Autodesk Inventor part; units mm, degrees
(part 2 of 3)
  line L954 (15.7927, 2.8054) -> (15.8047, 2.9296)
  line L955 (15.8047, 2.9296) -> (15.8214, 3.0524)
  line L956 (15.8214, 3.0524) -> (15.8318, 3.1132)
  line L957 (15.8318, 3.1132) -> (15.8442, 3.1734)
  line L958 (15.8442, 3.1734) -> (15.5913, 3.315)
  line L959 (15.5913, 3.315) -> (15.2554, 3.4241)
  line L960 (15.2554, 3.4241) -> (14.9676, 3.4583)
  line L961 (14.9676, 3.4583) -> (14.9422, 3.4023)
  line L962 (14.9422, 3.4023) -> (14.915, 3.3469)
  line L963 (14.915, 3.3469) -> (14.8562, 3.2378)
  line L964 (14.8562, 3.2378) -> (14.7929, 3.1303)
  line L965 (14.7929, 3.1303) -> (14.7259, 3.0241)
  line L966 (14.7259, 3.0241) -> (14.5818, 2.8156)
  line L967 (14.5818, 2.8156) -> (14.4261, 2.6115)
  line L968 (14.4261, 2.6115) -> (14.2601, 2.4115)
  line L969 (14.2601, 2.4115) -> (14.0847, 2.2154)
  line L970 (14.0847, 2.2154) -> (13.9004, 2.0233)
  line L971 (13.9004, 2.0233) -> (13.7077, 1.8349)
  line L972 (13.7077, 1.8349) -> (13.507, 1.6503)
  line L973 (13.507, 1.6503) -> (13.3514, 1.5144)
  line L974 (13.3514, 1.5144) -> (12.8549, 1.72)
  line L975 (12.8549, 1.72) -> (12.841, 1.9262)
  line L976 (12.841, 1.9262) -> (12.8296, 2.1986)
  line L977 (12.8296, 2.1986) -> (12.8265, 2.4681)
  line L978 (12.8265, 2.4681) -> (12.8321, 2.7343)
  line L979 (12.8321, 2.7343) -> (12.8466, 2.997)
  line L980 (12.8466, 2.997) -> (12.8707, 3.2557)
  line L981 (12.8707, 3.2557) -> (12.9049, 3.5101)
  line L982 (12.9049, 3.5101) -> (12.9505, 3.7595)
  line L983 (12.9505, 3.7595) -> (12.9781, 3.882)
  line L984 (12.9781, 3.882) -> (13.0095, 4.0027)
  line L985 (13.0095, 4.0027) -> (13.0451, 4.1215)
  line L986 (13.0451, 4.1215) -> (13.0649, 4.1799)
  line L987 (13.0649, 4.1799) -> (13.0865, 4.2374)
  line L988 (13.0865, 4.2374) -> (12.8589, 4.4167)
  line L989 (12.8589, 4.4167) -> (12.5442, 4.5771)
  line L990 (12.5442, 4.5771) -> (12.2654, 4.6558)
  line L991 (12.2654, 4.6558) -> (12.2315, 4.6045)
  line L992 (12.2315, 4.6045) -> (12.1959, 4.5541)
  line L993 (12.1959, 4.5541) -> (12.1208, 4.4555)
  line L994 (12.1208, 4.4555) -> (12.0415, 4.3592)
  line L995 (12.0415, 4.3592) -> (11.9586, 4.2649)
  line L996 (11.9586, 4.2649) -> (11.7837, 4.0814)
  line L997 (11.7837, 4.0814) -> (11.5981, 3.9042)
  line L998 (11.5981, 3.9042) -> (11.4028, 3.7326)
  line L999 (11.4028, 3.7326) -> (11.1989, 3.5664)
  line L1000 (11.1989, 3.5664) -> (10.9868, 3.4055)
  line L1001 (10.9868, 3.4055) -> (10.7669, 3.2496)
  line L1002 (10.7669, 3.2496) -> (10.5398, 3.0987)
  line L1003 (10.5398, 3.0987) -> (10.3649, 2.9888)
  line L1004 (10.3649, 2.9888) -> (9.9067, 3.2695)
  line L1005 (9.9067, 3.2695) -> (9.9252, 3.4753)
  line L1006 (9.9252, 3.4753) -> (9.9566, 3.7462)
  line L1007 (9.9566, 3.7462) -> (9.9957, 4.0128)
  line L1008 (9.9957, 4.0128) -> (10.0428, 4.2749)
  line L1009 (10.0428, 4.2749) -> (10.0983, 4.532)
  line L1010 (10.0983, 4.532) -> (10.1625, 4.7839)
  line L1011 (10.1625, 4.7839) -> (10.2362, 5.0298)
  line L1012 (10.2362, 5.0298) -> (10.3202, 5.2689)
  line L1013 (10.3202, 5.2689) -> (10.3666, 5.3856)
  line L1014 (10.3666, 5.3856) -> (10.4164, 5.5)
  line L1015 (10.4164, 5.5) -> (10.4702, 5.6116)
  line L1016 (10.4702, 5.6116) -> (10.499, 5.6662)
  line L1017 (10.499, 5.6662) -> (10.5293, 5.7197)
  line L1018 (10.5293, 5.7197) -> (10.3326, 5.9324)
  line L1019 (10.3326, 5.9324) -> (10.0468, 6.14)
  line L1020 (10.0468, 6.14) -> (9.7837, 6.2614)
  line L1021 (9.7837, 6.2614) -> (9.7422, 6.216)
  line L1022 (9.7422, 6.216) -> (9.6992, 6.1718)
  line L1023 (9.6992, 6.1718) -> (9.6096, 6.0862)
  line L1024 (9.6096, 6.0862) -> (9.5162, 6.0035)
  line L1025 (9.5162, 6.0035) -> (9.4196, 5.9233)
  line L1026 (9.4196, 5.9233) -> (9.2181, 5.7694)
  line L1027 (9.2181, 5.7694) -> (9.007, 5.6234)
  line L1028 (9.007, 5.6234) -> (8.7874, 5.4845)
  line L1029 (8.7874, 5.4845) -> (8.5599, 5.3523)
  line L1030 (8.5599, 5.3523) -> (8.3252, 5.2265)
  line L1031 (8.3252, 5.2265) -> (8.0837, 5.1069)
  line L1032 (8.0837, 5.1069) -> (7.8358, 4.9934)
  line L1033 (7.8358, 4.9934) -> (7.6459, 4.9122)
  line L1034 (7.6459, 4.9122) -> (7.2372, 5.2611)
  line L1035 (7.2372, 5.2611) -> (7.2877, 5.4615)
  line L1036 (7.2877, 5.4615) -> (7.361, 5.7241)
  line L1037 (7.361, 5.7241) -> (7.4414, 5.9813)
  line L1038 (7.4414, 5.9813) -> (7.5289, 6.2328)
  line L1039 (7.5289, 6.2328) -> (7.6239, 6.4781)
  line L1040 (7.6239, 6.4781) -> (7.7268, 6.7168)
  line L1041 (7.7268, 6.7168) -> (7.838, 6.9482)
  line L1042 (7.838, 6.9482) -> (7.9584, 7.1712)
  line L1043 (7.9584, 7.1712) -> (8.0225, 7.2792)
  line L1044 (8.0225, 7.2792) -> (8.0896, 7.3844)
  line L1045 (8.0896, 7.3844) -> (8.1602, 7.4863)
  line L1046 (8.1602, 7.4863) -> (8.1971, 7.5357)
  line L1047 (8.1971, 7.5357) -> (8.2354, 7.5837)
  line L1048 (8.2354, 7.5837) -> (8.0744, 7.8246)
  line L1049 (8.0744, 7.8246) -> (7.8246, 8.0744)
  line L1050 (7.8246, 8.0744) -> (7.5837, 8.2354)
  line L1051 (7.5837, 8.2354) -> (7.5357, 8.1971)
  line L1052 (7.5357, 8.1971) -> (7.4863, 8.1602)
  line L1053 (7.4863, 8.1602) -> (7.3844, 8.0896)
  line L1054 (7.3844, 8.0896) -> (7.2792, 8.0225)
  line L1055 (7.2792, 8.0225) -> (7.1712, 7.9584)
  line L1056 (7.1712, 7.9584) -> (6.9482, 7.838)
  line L1057 (6.9482, 7.838) -> (6.7168, 7.7268)
  line L1058 (6.7168, 7.7268) -> (6.4781, 7.6239)
  line L1059 (6.4781, 7.6239) -> (6.2328, 7.5289)
  line L1060 (6.2328, 7.5289) -> (5.9813, 7.4414)
  line L1061 (5.9813, 7.4414) -> (5.7241, 7.361)
  line L1062 (5.7241, 7.361) -> (5.4615, 7.2877)
  line L1063 (5.4615, 7.2877) -> (5.2611, 7.2372)
  line L1064 (5.2611, 7.2372) -> (4.9122, 7.6459)
  line L1065 (4.9122, 7.6459) -> (4.9934, 7.8358)
  line L1066 (4.9934, 7.8358) -> (5.1069, 8.0837)
  line L1067 (5.1069, 8.0837) -> (5.2265, 8.3252)
  line L1068 (5.2265, 8.3252) -> (5.3523, 8.5599)
  line L1069 (5.3523, 8.5599) -> (5.4845, 8.7874)
  line L1070 (5.4845, 8.7874) -> (5.6234, 9.007)
  line L1071 (5.6234, 9.007) -> (5.7694, 9.2181)
  line L1072 (5.7694, 9.2181) -> (5.9233, 9.4196)
  line L1073 (5.9233, 9.4196) -> (6.0035, 9.5162)
  line L1074 (6.0035, 9.5162) -> (6.0862, 9.6096)
  line L1075 (6.0862, 9.6096) -> (6.1718, 9.6992)
  line L1076 (6.1718, 9.6992) -> (6.216, 9.7422)
  line L1077 (6.216, 9.7422) -> (6.2614, 9.7837)
  line L1078 (6.2614, 9.7837) -> (6.14, 10.0468)
  line L1079 (6.14, 10.0468) -> (5.9324, 10.3326)
  line L1080 (5.9324, 10.3326) -> (5.7197, 10.5293)
  line L1081 (5.7197, 10.5293) -> (5.6662, 10.499)
  line L1082 (5.6662, 10.499) -> (5.6116, 10.4702)
  line L1083 (5.6116, 10.4702) -> (5.5, 10.4164)
  line L1084 (5.5, 10.4164) -> (5.3856, 10.3666)
  line L1085 (5.3856, 10.3666) -> (5.2689, 10.3202)
  line L1086 (5.2689, 10.3202) -> (5.0298, 10.2362)
  line L1087 (5.0298, 10.2362) -> (4.7839, 10.1625)
  line L1088 (4.7839, 10.1625) -> (4.532, 10.0983)
  line L1089 (4.532, 10.0983) -> (4.2749, 10.0428)
  line L1090 (4.2749, 10.0428) -> (4.0128, 9.9957)
  line L1091 (4.0128, 9.9957) -> (3.7462, 9.9566)
  line L1092 (3.7462, 9.9566) -> (3.4753, 9.9252)
  line L1093 (3.4753, 9.9252) -> (3.2695, 9.9067)
  line L1094 (3.2695, 9.9067) -> (2.9888, 10.3649)
  line L1095 (2.9888, 10.3649) -> (3.0987, 10.5398)
  line L1096 (3.0987, 10.5398) -> (3.2496, 10.7669)
  line L1097 (3.2496, 10.7669) -> (3.4055, 10.9868)
  line L1098 (3.4055, 10.9868) -> (3.5664, 11.1989)
  line L1099 (3.5664, 11.1989) -> (3.7326, 11.4028)
  line L1100 (3.7326, 11.4028) -> (3.9042, 11.5981)
  line L1101 (3.9042, 11.5981) -> (4.0814, 11.7837)
  line L1102 (4.0814, 11.7837) -> (4.2649, 11.9586)
  line L1103 (4.2649, 11.9586) -> (4.3592, 12.0415)
  line L1104 (4.3592, 12.0415) -> (4.4555, 12.1208)
  line L1105 (4.4555, 12.1208) -> (4.5541, 12.1959)
  line L1106 (4.5541, 12.1959) -> (4.6045, 12.2315)
  line L1107 (4.6045, 12.2315) -> (4.6558, 12.2654)
  line L1108 (4.6558, 12.2654) -> (4.5771, 12.5442)
  line L1109 (4.5771, 12.5442) -> (4.4167, 12.8589)
  line L1110 (4.4167, 12.8589) -> (4.2374, 13.0865)
  line L1111 (4.2374, 13.0865) -> (4.1799, 13.0649)
  line L1112 (4.1799, 13.0649) -> (4.1215, 13.0451)
  line L1113 (4.1215, 13.0451) -> (4.0027, 13.0095)
  line L1114 (4.0027, 13.0095) -> (3.882, 12.9781)
  line L1115 (3.882, 12.9781) -> (3.7595, 12.9505)
  line L1116 (3.7595, 12.9505) -> (3.5101, 12.9049)
  line L1117 (3.5101, 12.9049) -> (3.2557, 12.8707)
  line L1118 (3.2557, 12.8707) -> (2.997, 12.8466)
  line L1119 (2.997, 12.8466) -> (2.7343, 12.8321)
  line L1120 (2.7343, 12.8321) -> (2.4681, 12.8265)
  line L1121 (2.4681, 12.8265) -> (2.1986, 12.8296)
  line L1122 (2.1986, 12.8296) -> (1.9262, 12.841)
  line L1123 (1.9262, 12.841) -> (1.72, 12.8549)
  line L1124 (1.72, 12.8549) -> (1.5144, 13.3514)
  line L1125 (1.5144, 13.3514) -> (1.6503, 13.507)
  line L1126 (1.6503, 13.507) -> (1.8349, 13.7077)
  line L1127 (1.8349, 13.7077) -> (2.0233, 13.9004)
  line L1128 (2.0233, 13.9004) -> (2.2154, 14.0847)
  line L1129 (2.2154, 14.0847) -> (2.4115, 14.2601)
  line L1130 (2.4115, 14.2601) -> (2.6115, 14.4261)
  line L1131 (2.6115, 14.4261) -> (2.8156, 14.5818)
  line L1132 (2.8156, 14.5818) -> (3.0241, 14.7259)
  line L1133 (3.0241, 14.7259) -> (3.1303, 14.7929)
  line L1134 (3.1303, 14.7929) -> (3.2378, 14.8562)
  line L1135 (3.2378, 14.8562) -> (3.3469, 14.915)
  line L1136 (3.3469, 14.915) -> (3.4023, 14.9422)
  line L1137 (3.4023, 14.9422) -> (3.4583, 14.9676)
  line L1138 (3.4583, 14.9676) -> (3.4241, 15.2554)
  line L1139 (3.4241, 15.2554) -> (3.315, 15.5913)
  line L1140 (3.315, 15.5913) -> (3.1734, 15.8442)
  line L1141 (3.1734, 15.8442) -> (3.1132, 15.8318)
  line L1142 (3.1132, 15.8318) -> (3.0524, 15.8214)
  line L1143 (3.0524, 15.8214) -> (2.9296, 15.8047)
  line L1144 (2.9296, 15.8047) -> (2.8054, 15.7927)
  line L1145 (2.8054, 15.7927) -> (2.6801, 15.7846)
  line L1146 (2.6801, 15.7846) -> (2.4267, 15.7786)
  line L1147 (2.4267, 15.7786) -> (2.1701, 15.7845)
  line L1148 (2.1701, 15.7845) -> (1.9107, 15.8012)
  line L1149 (1.9107, 15.8012) -> (1.649, 15.828)
  line L1150 (1.649, 15.828) -> (1.3852, 15.8641)
  line L1151 (1.3852, 15.8641) -> (1.1195, 15.9093)
  line L1152 (1.1195, 15.9093) -> (0.8522, 15.9632)
  line L1153 (0.8522, 15.9632) -> (0.6508, 16.0092)
  line L1154 (0.6508, 16.0092) -> (0.5254, 16.5317)
  line L1155 (0.5254, 16.5317) -> (0.684, 16.6641)
  line L1156 (0.684, 16.6641) -> (0.8977, 16.8335)
  line L1157 (0.8977, 16.8335) -> (1.1139, 16.9944)
  line L1158 (1.1139, 16.9944) -> (1.3325, 17.1463)
  line L1159 (1.3325, 17.1463) -> (1.5536, 17.289)
  line L1160 (1.5536, 17.289) -> (1.777, 17.4216)
  line L1161 (1.777, 17.4216) -> (2.003, 17.5434)
  line L1162 (2.003, 17.5434) -> (2.2315, 17.6531)
  line L1163 (2.2315, 17.6531) -> (2.3469, 17.7028)
  line L1164 (2.3469, 17.7028) -> (2.463, 17.7484)
  line L1165 (2.463, 17.7484) -> (2.58, 17.7894)
  line L1166 (2.58, 17.7894) -> (2.6389, 17.8076)
  line L1167 (2.6389, 17.8076) -> (2.6981, 17.824)
  line L1168 (2.6981, 17.824) -> (2.7094, 18.1135)
  line L1169 (2.7094, 18.1135) -> (2.6542, 18.4624)
  line L1170 (2.6542, 18.4624) -> (2.554, 18.7343)
  line L1171 (2.554, 18.7343) -> (2.4925, 18.7315)
  line L1172 (2.4925, 18.7315) -> (2.4309, 18.7307)
  line L1173 (2.4309, 18.7307) -> (2.3069, 18.7335)
  line L1174 (2.3069, 18.7335) -> (2.1824, 18.741)
  line L1175 (2.1824, 18.741) -> (2.0574, 18.7526)
  line L1176 (2.0574, 18.7526) -> (1.8061, 18.7863)
  line L1177 (1.8061, 18.7863) -> (1.5536, 18.8323)
  line L1178 (1.5536, 18.8323) -> (1.3001, 18.8894)
  line L1179 (1.3001, 18.8894) -> (1.0457, 18.9568)
  line L1180 (1.0457, 18.9568) -> (0.7908, 19.0338)
  line L1181 (0.7908, 19.0338) -> (0.5355, 19.1199)
  line L1182 (0.5355, 19.1199) -> (0.2799, 19.215)
  line L1183 (0.2799, 19.215) -> (0.0882, 19.2919)
  line L1184 (0.0882, 19.2919) -> (0.046, 19.8276)
  line L1185 (0.046, 19.8276) -> (0.2234, 19.9336)
  line L1186 (0.2234, 19.9336) -> (0.461, 20.0674)
  line L1187 (0.461, 20.0674) -> (0.6996, 20.1925)
  line L1188 (0.6996, 20.1925) -> (0.9394, 20.3084)
  line L1189 (0.9394, 20.3084) -> (1.18, 20.4147)
  line L1190 (1.18, 20.4147) -> (1.4215, 20.5108)
  line L1191 (1.4215, 20.5108) -> (1.6637, 20.5957)
  line L1192 (1.6637, 20.5957) -> (1.9066, 20.6683)
  line L1193 (1.9066, 20.6683) -> (2.0283, 20.6993)
  line L1194 (2.0283, 20.6993) -> (2.1501, 20.7262)
  line L1195 (2.1501, 20.7262) -> (2.2721, 20.7484)
  line L1196 (2.2721, 20.7484) -> (2.3331, 20.7572)
  line L1197 (2.3331, 20.7572) -> (2.3942, 20.7641)
  line L1198 (2.3942, 20.7641) -> (2.4506, 21.0483)
  line L1199 (2.4506, 21.0483) -> (2.4506, 21.4015)
  circle A0 centre (21.2249, 21.2249) radius 0.5
  line L1200 (0.0671, 22.8901) -> (42.3827, 19.5598) construction
  line L1201 (19.5598, 0.0671) -> (22.8901, 42.3827) construction
  point P0 (21.2249, 21.2249)
derived "gear_central_part_30.ipt"
sketch "Sketch9" plane through (0, 0, 0) normal (0, 1, 0) x (-1, 0, 0)
  circle A0 centre (0, 0) radius 15
  arc A1 (4.5, -13.2571) -> (5.5, -12.8744) centre (0, 0) ccw
  line L0 (0, 0) -> (20.2233, 0) construction
  line L1 (0, 0) -> (0, -27.3647) construction
  line L2 (0.2121, 2.4395) -> (2.4395, 0.2121)
  line L3 (2.4395, -0.2121) -> (0.2121, -2.4395)
  line L4 (-0.2121, -2.4395) -> (-2.4395, -0.2121)
  line L5 (-2.4395, 0.2121) -> (-0.2121, 2.4395)
  line L6 (0, 2.6517) -> (0, -2.6517) construction
  line L7 (2.6517, 0) -> (-2.6517, 0) construction
  arc A2 (2.4395, -0.2121) -> (2.4395, 0.2121) centre (2.2274, 0) ccw
  arc A3 (-0.2121, -2.4395) -> (0.2121, -2.4395) centre (0, -2.2274) ccw
  arc A4 (-2.4395, 0.2121) -> (-2.4395, -0.2121) centre (-2.2274, 0) ccw
  arc A5 (0.2121, 2.4395) -> (-0.2121, 2.4395) centre (0, 2.2274) ccw
  line L8 (-3.1466, -0.9192) -> (-0.9192, -3.1466)
  arc A6 (-0.9192, -3.1466) -> (0.9192, -3.1466) centre (0, -2.2274) ccw
  line L9 (0.9192, -3.1466) -> (3.1466, -0.9192)
  arc A7 (3.1466, -0.9192) -> (3.1466, 0.9192) centre (2.2274, 0) ccw
  line L10 (3.1466, 0.9192) -> (0.9192, 3.1466)
  arc A8 (0.9192, 3.1466) -> (-0.9192, 3.1466) centre (0, 2.2274) ccw
  line L11 (-0.9192, 3.1466) -> (-3.1466, 0.9192)
  arc A9 (-3.1466, 0.9192) -> (-3.1466, -0.9192) centre (-2.2274, 0) ccw
  circle A10 centre (10, 0) radius 2.5
  arc A11 (13.4641, -0.5) -> (9.5, -3.4641) centre (10, 0) ccw
  line L12 (3.4274, -0.5) -> (6.5359, -0.5)
  line L13 (3.4274, 0.5) -> (6.5359, 0.5)
  line L14 (13.9911, 0.5) -> (13.4641, 0.5)
  line L15 (13.9911, -0.5) -> (13.4641, -0.5)
  line L16 (0, -5) -> (13.0767, -5) construction
  line L17 (0, -4.5) -> (13.2571, -4.5)
  line L18 (0, -5.5) -> (12.8744, -5.5)
  line L19 (5, 0) -> (5, -13.0767) construction
  line L20 (5.5, 12.8744) -> (5.5, -12.8744)
  line L21 (4.5, 13.2571) -> (4.5, -13.2571)
  arc A12 (0, -14) -> (4.5, -13.2571) centre (0, 0) ccw
  arc A13 (5.5, -12.8744) -> (12.8744, -5.5) centre (0, 0) ccw
  arc A14 (12.8744, -5.5) -> (13.2571, -4.5) centre (0, 0) ccw
  arc A15 (13.2571, -4.5) -> (13.9911, -0.5) centre (0, 0) ccw
  arc A16 (13.9911, -0.5) -> (13.9911, 0.5) centre (0, 0) ccw
  arc A17 (13.9911, 0.5) -> (5.5, 12.8744) centre (0, 0) ccw
  line L22 (0.5, -4.5) -> (0.5, -5.5)
  line L23 (10, 0) -> (10, -4.5) construction
  line L24 (10.5, -3.4641) -> (10.5, -4.5)
  line L25 (9.5, -3.4641) -> (9.5, -4.5)
  arc A18 (10.5, -3.4641) -> (13.4641, -0.5) centre (10, 0) ccw
  arc A19 (9.5, -3.4641) -> (10.5, -3.4641) centre (10, 0) ccw
  arc A20 (10.5, 3.4641) -> (9.5, 3.4641) centre (10, 0) ccw
  line L26 (0, -4.5) -> (0, -5.5)
  arc A21 (4.5, 13.2571) -> (0, -14) centre (0, 0) ccw
  arc A22 (5.5, 12.8744) -> (4.5, 13.2571) centre (0, 0) ccw
  line L27 (0, 4.5) -> (0, 5.5)
  line L28 (9.5, 3.4641) -> (9.5, 4.5)
  arc A23 (10.5, 3.4641) -> (9.5, 3.4641) centre (10, 0) ccw
  line L29 (0.5, 4.5) -> (0.5, 5.5)
  line L30 (0, 4.5) -> (13.2571, 4.5)
  line L31 (0, 5) -> (13.0767, 5) construction
  line L32 (0, 5.5) -> (12.8744, 5.5)
  arc A24 (13.2571, 4.5) -> (12.8744, 5.5) centre (0, 0) ccw
  line L33 (10.5, 3.4641) -> (10.5, 4.5)
  arc A25 (2.4395, -0.2121) -> (2.4395, 0.2121) centre (2.2274, 0) ccw
  line L34 (0.2121, 2.4395) -> (2.4395, 0.2121)
  line L35 (0.9192, -3.1466) -> (3.1466, -0.9192)
  arc A26 (0.2121, 2.4395) -> (-0.2121, 2.4395) centre (0, 2.2274) ccw
  line L36 (2.4395, -0.2121) -> (0.2121, -2.4395)
  line L37 (0, 2.6517) -> (0, -2.6517) construction
  line L38 (-2.4395, 0.2121) -> (-0.2121, 2.4395)
  line L39 (-2.6517, 0) -> (2.6517, 0) construction
  arc A27 (-0.2121, -2.4395) -> (0.2121, -2.4395) centre (0, -2.2274) ccw
  line L40 (-0.2121, -2.4395) -> (-2.4395, -0.2121)
  arc A28 (3.1466, -0.9192) -> (3.1466, 0.9192) centre (2.2274, 0) ccw
  line L41 (3.1466, 0.9192) -> (0.9192, 3.1466)
  line L42 (4.5, 0.5) -> (5.5, 0.5)
  line L43 (4.5, 0) -> (5.5, 0)
  line L44 (-13.2571, 4.5) -> (13.2571, 4.5)
  line L45 (0, 5) -> (13.0767, 5) construction
  arc A29 (14, 0) -> (13.2571, 4.5) centre (0, 0) ccw
  arc A30 (-0.9192, -3.1466) -> (0.9192, -3.1466) centre (0, -2.2274) ccw
  line L46 (-3.1466, -0.9192) -> (-0.9192, -3.1466)
  arc A31 (-12.8744, 5.5) -> (-13.2571, 4.5) centre (0, 0) ccw
  circle A32 centre (0, 10) radius 2.5
  arc A33 (0.5, 13.4641) -> (3.4641, 9.5) centre (0, 10) ccw
  line L47 (0.5, 3.4274) -> (0.5, 6.5359)
  line L48 (-0.5, 3.4274) -> (-0.5, 6.5359)
  arc A34 (3.4641, 10.5) -> (0.5, 13.4641) centre (0, 10) ccw
  line L49 (0, 10) -> (4.5, 10) construction
  line L50 (0.5, 13.9911) -> (0.5, 13.4641)
  arc A35 (4.5, 13.2571) -> (0.5, 13.9911) centre (0, 0) ccw
  line L51 (-12.8744, 5.5) -> (12.8744, 5.5)
  arc A36 (0.5, 13.9911) -> (-0.5, 13.9911) centre (0, 0) ccw
  line L52 (-0.5, 13.9911) -> (-0.5, 13.4641)
  arc A37 (13.2571, 4.5) -> (12.8744, 5.5) centre (0, 0) ccw
  arc A38 (3.4641, 9.5) -> (3.4641, 10.5) centre (0, 10) ccw
  line L53 (3.4641, 9.5) -> (4.5, 9.5)
  line L54 (3.4641, 10.5) -> (4.5, 10.5)
  arc A39 (5.5, 12.8744) -> (4.5, 13.2571) centre (0, 0) ccw
  line L55 (4.5, 0) -> (4.5, 13.2571)
  line L56 (5, 0) -> (5, 13.0767) construction
  line L57 (5.5, 0) -> (5.5, 12.8744)
  arc A40 (12.8744, 5.5) -> (5.5, 12.8744) centre (0, 0) ccw
  line L58 (-0.9192, 3.1466) -> (-3.1466, 0.9192)
  arc A41 (-3.4641, 10.5) -> (-3.4641, 9.5) centre (0, 10) ccw
  arc A42 (-3.4641, 10.5) -> (-3.4641, 9.5) centre (0, 10) ccw
  line L59 (-3.4641, 10.5) -> (-4.5, 10.5)
  line L60 (-4.5, 0) -> (-4.5, 13.2571)
  line L61 (-5, 0) -> (-5, 13.0767) construction
  line L62 (-5.5, 0) -> (-5.5, 12.8744)
  arc A43 (-4.5, 13.2571) -> (-5.5, 12.8744) centre (0, 0) ccw
  arc A44 (-0.5, 13.9911) -> (-12.8744, 5.5) centre (0, 0) ccw
  line L63 (-3.4641, 9.5) -> (-4.5, 9.5)
  line L64 (-4.5, 0.5) -> (-5.5, 0.5)
  line L65 (-4.5, 0) -> (-5.5, 0)
  arc A45 (-2.4395, 0.2121) -> (-2.4395, -0.2121) centre (-2.2274, 0) ccw
  arc A46 (-3.1466, 0.9192) -> (-3.1466, -0.9192) centre (-2.2274, 0) ccw
  arc A47 (0.9192, 3.1466) -> (-0.9192, 3.1466) centre (0, 2.2274) ccw
  arc A48 (0.2121, 2.4395) -> (-0.2121, 2.4395) centre (0, 2.2274) ccw
  line L66 (-2.4395, 0.2121) -> (-0.2121, 2.4395)
  line L67 (3.1466, 0.9192) -> (0.9192, 3.1466)
  arc A49 (-2.4395, 0.2121) -> (-2.4395, -0.2121) centre (-2.2274, 0) ccw
  line L68 (0.2121, 2.4395) -> (2.4395, 0.2121)
  line L69 (-2.6517, 0) -> (2.6517, 0) construction
  line L70 (-0.2121, -2.4395) -> (-2.4395, -0.2121)
  line L71 (0, -2.6517) -> (0, 2.6517) construction
  arc A50 (2.4395, -0.2121) -> (2.4395, 0.2121) centre (2.2274, 0) ccw
  line L72 (2.4395, -0.2121) -> (0.2121, -2.4395)
  arc A51 (0.9192, 3.1466) -> (-0.9192, 3.1466) centre (0, 2.2274) ccw
  line L73 (-0.9192, 3.1466) -> (-3.1466, 0.9192)
  line L74 (-0.5, 4.5) -> (-0.5, 5.5)
  line L75 (0, 4.5) -> (0, 5.5)
  line L76 (-4.5, -13.2571) -> (-4.5, 13.2571)
  line L77 (-5, 0) -> (-5, 13.0767) construction
  arc A52 (0, 14) -> (-4.5, 13.2571) centre (0, 0) ccw
  arc A53 (3.1466, -0.9192) -> (3.1466, 0.9192) centre (2.2274, 0) ccw
  line L78 (0.9192, -3.1466) -> (3.1466, -0.9192)
  arc A54 (-5.5, -12.8744) -> (-4.5, -13.2571) centre (0, 0) ccw
  circle A55 centre (-10, 0) radius 2.5
  arc A56 (-13.4641, 0.5) -> (-9.5, 3.4641) centre (-10, 0) ccw
  line L79 (-3.4274, 0.5) -> (-6.5359, 0.5)
  line L80 (-3.4274, -0.5) -> (-6.5359, -0.5)
  arc A57 (-10.5, 3.4641) -> (-13.4641, 0.5) centre (-10, 0) ccw
  line L81 (-10, 0) -> (-10, 4.5) construction
  line L82 (-13.9911, 0.5) -> (-13.4641, 0.5)
  arc A58 (-13.2571, 4.5) -> (-13.9911, 0.5) centre (0, 0) ccw
  line L83 (-5.5, -12.8744) -> (-5.5, 12.8744)
  arc A59 (-13.9911, 0.5) -> (-13.9911, -0.5) centre (0, 0) ccw
  line L84 (-13.9911, -0.5) -> (-13.4641, -0.5)
  arc A60 (-4.5, 13.2571) -> (-5.5, 12.8744) centre (0, 0) ccw
  arc A61 (-9.5, 3.4641) -> (-10.5, 3.4641) centre (-10, 0) ccw
  line L85 (-9.5, 3.4641) -> (-9.5, 4.5)
  line L86 (-10.5, 3.4641) -> (-10.5, 4.5)
  arc A62 (-12.8744, 5.5) -> (-13.2571, 4.5) centre (0, 0) ccw
  line L87 (0, 4.5) -> (-13.2571, 4.5)
  line L88 (0, 5) -> (-13.0767, 5) construction
  line L89 (0, 5.5) -> (-12.8744, 5.5)
  arc A63 (-5.5, 12.8744) -> (-12.8744, 5.5) centre (0, 0) ccw
  line L90 (-3.1466, -0.9192) -> (-0.9192, -3.1466)
  arc A64 (-10.5, -3.4641) -> (-9.5, -3.4641) centre (-10, 0) ccw
  arc A65 (-10.5, -3.4641) -> (-9.5, -3.4641) centre (-10, 0) ccw
  line L91 (-10.5, -3.4641) -> (-10.5, -4.5)
  line L92 (0, -4.5) -> (-13.2571, -4.5)
  line L93 (0, -5) -> (-13.0767, -5) construction
  line L94 (0, -5.5) -> (-12.8744, -5.5)
  arc A66 (-13.2571, -4.5) -> (-12.8744, -5.5) centre (0, 0) ccw
  arc A67 (-13.9911, -0.5) -> (-5.5, -12.8744) centre (0, 0) ccw
  line L95 (-9.5, -3.4641) -> (-9.5, -4.5)
  line L96 (-0.5, -4.5) -> (-0.5, -5.5)
  line L97 (0, -4.5) -> (0, -5.5)
  arc A68 (-0.2121, -2.4395) -> (0.2121, -2.4395) centre (0, -2.2274) ccw
  arc A69 (-0.9192, -3.1466) -> (0.9192, -3.1466) centre (0, -2.2274) ccw
  arc A70 (-3.1466, 0.9192) -> (-3.1466, -0.9192) centre (-2.2274, 0) ccw
  arc A71 (-2.4395, 0.2121) -> (-2.4395, -0.2121) centre (-2.2274, 0) ccw
  line L98 (-0.2121, -2.4395) -> (-2.4395, -0.2121)
  line L99 (-0.9192, 3.1466) -> (-3.1466, 0.9192)
  arc A72 (-0.2121, -2.4395) -> (0.2121, -2.4395) centre (0, -2.2274) ccw
  line L100 (-2.4395, 0.2121) -> (-0.2121, 2.4395)
  line L101 (0, -2.6517) -> (0, 2.6517) construction
  line L102 (2.4395, -0.2121) -> (0.2121, -2.4395)
  line L103 (2.6517, 0) -> (-2.6517, 0) construction
  arc A73 (0.2121, 2.4395) -> (-0.2121, 2.4395) centre (0, 2.2274) ccw
  line L104 (0.2121, 2.4395) -> (2.4395, 0.2121)
  arc A74 (-3.1466, 0.9192) -> (-3.1466, -0.9192) centre (-2.2274, 0) ccw
  line L105 (-3.1466, -0.9192) -> (-0.9192, -3.1466)
  line L106 (-4.5, -0.5) -> (-5.5, -0.5)
  line L107 (-4.5, 0) -> (-5.5, 0)
  line L108 (13.2571, -4.5) -> (-13.2571, -4.5)
  line L109 (0, -5) -> (-13.0767, -5) construction
  arc A75 (-14, 0) -> (-13.2571, -4.5) centre (0, 0) ccw
  arc A76 (0.9192, 3.1466) -> (-0.9192, 3.1466) centre (0, 2.2274) ccw
  line L110 (3.1466, 0.9192) -> (0.9192, 3.1466)
  arc A77 (12.8744, -5.5) -> (13.2571, -4.5) centre (0, 0) ccw
  circle A78 centre (0, -10) radius 2.5
  arc A79 (-0.5, -13.4641) -> (-3.4641, -9.5) centre (0, -10) ccw
  line L111 (-0.5, -3.4274) -> (-0.5, -6.5359)
  line L112 (0.5, -3.4274) -> (0.5, -6.5359)
  arc A80 (-3.4641, -10.5) -> (-0.5, -13.4641) centre (0, -10) ccw
  line L113 (0, -10) -> (-4.5, -10) construction
  line L114 (-0.5, -13.9911) -> (-0.5, -13.4641)
  arc A81 (-4.5, -13.2571) -> (-0.5, -13.9911) centre (0, 0) ccw
  line L115 (12.8744, -5.5) -> (-12.8744, -5.5)
  arc A82 (-0.5, -13.9911) -> (0.5, -13.9911) centre (0, 0) ccw
  line L116 (0.5, -13.9911) -> (0.5, -13.4641)
  arc A83 (-13.2571, -4.5) -> (-12.8744, -5.5) centre (0, 0) ccw
  arc A84 (-3.4641, -9.5) -> (-3.4641, -10.5) centre (0, -10) ccw
  line L117 (-3.4641, -9.5) -> (-4.5, -9.5)
  line L118 (-3.4641, -10.5) -> (-4.5, -10.5)
  arc A85 (-5.5, -12.8744) -> (-4.5, -13.2571) centre (0, 0) ccw
  line L119 (-4.5, 0) -> (-4.5, -13.2571)
  line L120 (-5, 0) -> (-5, -13.0767) construction
  line L121 (-5.5, 0) -> (-5.5, -12.8744)
  arc A86 (-12.8744, -5.5) -> (-5.5, -12.8744) centre (0, 0) ccw
  line L122 (0.9192, -3.1466) -> (3.1466, -0.9192)
  arc A87 (3.4641, -10.5) -> (3.4641, -9.5) centre (0, -10) ccw
  arc A88 (3.4641, -10.5) -> (3.4641, -9.5) centre (0, -10) ccw
  line L123 (3.4641, -10.5) -> (4.5, -10.5)
  line L124 (4.5, 0) -> (4.5, -13.2571)
  line L125 (5, 0) -> (5, -13.0767) construction
  line L126 (5.5, 0) -> (5.5, -12.8744)
  arc A89 (4.5, -13.2571) -> (5.5, -12.8744) centre (0, 0) ccw
  arc A90 (0.5, -13.9911) -> (12.8744, -5.5) centre (0, 0) ccw
  line L127 (3.4641, -9.5) -> (4.5, -9.5)
  line L128 (4.5, -0.5) -> (5.5, -0.5)
  line L129 (4.5, 0) -> (5.5, 0)
  arc A91 (2.4395, -0.2121) -> (2.4395, 0.2121) centre (2.2274, 0) ccw
  arc A92 (3.1466, -0.9192) -> (3.1466, 0.9192) centre (2.2274, 0) ccw
  arc A93 (-0.9192, -3.1466) -> (0.9192, -3.1466) centre (0, -2.2274) ccw
  point P0 (0, 2.2274)
  point P1 (10, 4.5)
  point P2 (-4.5, 10)
  point P3 (-2.2274, 0)
  point P4 (-10, -4.5)
  point P5 (0, -2.2274)
  point P6 (4.5, -10)
  point P7 (2.2274, 0)
derived "Base_part.ipt"
sketch "Sketch10" plane through (0, 0, 0) normal (0, 1, 0) x (-1, 0, 0)
  line L0 (0, 0) -> (0, -14.7241) construction
  line L1 (0, 0) -> (-15.85, 0) construction
  circle A0 centre (0, 0) radius 15 projected
  arc A1 (-17.1952, 4.5) -> (-17.1952, -4.5) centre (0, 0) ccw
  line L2 (-13.9553, 5.5) -> (-16.9019, 5.5)
  line L3 (-14.3091, 4.5) -> (-17.1952, 4.5)
  line L4 (0, 5.5) -> (-12.8744, 5.5) construction
  line L5 (0, 4.5) -> (-13.2571, 4.5) construction
  line L6 (-14.3091, -4.5) -> (-17.1952, -4.5)
  line L7 (-13.9553, -5.5) -> (-16.9019, -5.5)
  line L8 (0, -4.5) -> (-13.2571, -4.5) construction
  line L9 (12.8744, -5.5) -> (-12.8744, -5.5) construction
  arc A2 (-16.9019, 5.5) -> (-17.1952, 4.5) centre (0, 0) ccw
  arc A3 (-17.1952, -4.5) -> (-16.9019, -5.5) centre (0, 0) ccw
  arc A4 (-16.9019, -5.5) -> (-16.9019, 5.5) centre (0, 0) ccw
  arc A5 (-13.9553, 5.5) -> (-14.3091, 4.5) centre (0, 0) ccw
  arc A6 (-14.3091, -4.5) -> (-13.9553, -5.5) centre (0, 0) ccw
  line L10 (-5.5, -13.9553) -> (-5.5, -16.9019)
  arc A7 (-5.5, -16.9019) -> (-4.5, -17.1952) centre (0, 0) ccw
  line L11 (-4.5, -14.3091) -> (-4.5, -17.1952)
  arc A8 (-5.5, -13.9553) -> (-4.5, -14.3091) centre (0, 0) ccw
  arc A9 (4.5, -14.3091) -> (5.5, -13.9553) centre (0, 0) ccw
  line L12 (5.5, -13.9553) -> (5.5, -16.9019)
  arc A10 (4.5, -17.1952) -> (5.5, -16.9019) centre (0, 0) ccw
  line L13 (4.5, -14.3091) -> (4.5, -17.1952)
  line L14 (13.9553, -5.5) -> (16.9019, -5.5)
  arc A11 (16.9019, -5.5) -> (17.1952, -4.5) centre (0, 0) ccw
  line L15 (14.3091, -4.5) -> (17.1952, -4.5)
  arc A12 (13.9553, -5.5) -> (14.3091, -4.5) centre (0, 0) ccw
  arc A13 (14.3091, 4.5) -> (13.9553, 5.5) centre (0, 0) ccw
  line L16 (13.9553, 5.5) -> (16.9019, 5.5)
  arc A14 (17.1952, 4.5) -> (16.9019, 5.5) centre (0, 0) ccw
  line L17 (14.3091, 4.5) -> (17.1952, 4.5)
  line L18 (5.5, 13.9553) -> (5.5, 16.9019)
  arc A15 (5.5, 16.9019) -> (4.5, 17.1952) centre (0, 0) ccw
  line L19 (4.5, 14.3091) -> (4.5, 17.1952)
  arc A16 (5.5, 13.9553) -> (4.5, 14.3091) centre (0, 0) ccw
  arc A17 (-4.5, 14.3091) -> (-5.5, 13.9553) centre (0, 0) ccw
  line L20 (-5.5, 13.9553) -> (-5.5, 16.9019)
  arc A18 (-4.5, 17.1952) -> (-5.5, 16.9019) centre (0, 0) ccw
  line L21 (-4.5, 14.3091) -> (-4.5, 17.1952)
  line L22 (-18.7303, -1.297) -> (-18.8088, -1.018)
  line L23 (-18.8088, -1.018) -> (-18.8703, -1.016)
  line L24 (-18.8703, -1.016) -> (-18.9318, -1.012)
  line L25 (-18.9318, -1.012) -> (-19.0551, -0.9995)
  line L26 (-19.0551, -0.9995) -> (-19.1787, -0.9822)
  line L27 (-19.1787, -0.9822) -> (-19.3024, -0.9608)
  line L28 (-19.3024, -0.9608) -> (-19.5502, -0.9075)
  line L29 (-19.5502, -0.9075) -> (-19.7984, -0.8418)
  line L30 (-19.7984, -0.8418) -> (-20.0467, -0.765)
  line L31 (-20.0467, -0.765) -> (-20.2949, -0.6779)
  line L32 (-20.2949, -0.6779) -> (-20.543, -0.5812)
  line L33 (-20.543, -0.5812) -> (-20.7908, -0.4752)
  line L34 (-20.7908, -0.4752) -> (-21.0381, -0.3604)
  line L35 (-21.0381, -0.3604) -> (-21.2232, -0.2687)
  line L36 (-21.2232, -0.2687) -> (-21.2232, 0.2687)
  line L37 (-21.2232, 0.2687) -> (-21.0381, 0.3604)
  line L38 (-21.0381, 0.3604) -> (-20.7908, 0.4752)
  line L39 (-20.7908, 0.4752) -> (-20.543, 0.5812)
  line L40 (-20.543, 0.5812) -> (-20.2949, 0.6779)
  line L41 (-20.2949, 0.6779) -> (-20.0467, 0.765)
  line L42 (-20.0467, 0.765) -> (-19.7984, 0.8418)
  line L43 (-19.7984, 0.8418) -> (-19.5502, 0.9075)
  line L44 (-19.5502, 0.9075) -> (-19.3024, 0.9608)
  line L45 (-19.3024, 0.9608) -> (-19.1787, 0.9822)
  line L46 (-19.1787, 0.9822) -> (-19.0551, 0.9995)
  line L47 (-19.0551, 0.9995) -> (-18.9318, 1.012)
  line L48 (-18.9318, 1.012) -> (-18.8703, 1.016)
  line L49 (-18.8703, 1.016) -> (-18.8088, 1.018)
  line L50 (-18.8088, 1.018) -> (-18.7302, 1.297)
  line L51 (-18.7302, 1.297) -> (-18.7025, 1.6491)
  line L52 (-18.7025, 1.6491) -> (-18.7365, 1.9368)
  line L53 (-18.7365, 1.9368) -> (-18.7969, 1.9485)
  line L54 (-18.7969, 1.9485) -> (-18.857, 1.9621)
  line L55 (-18.857, 1.9621) -> (-18.9769, 1.9937)
  line L56 (-18.9769, 1.9937) -> (-19.0962, 2.0301)
  line L57 (-19.0962, 2.0301) -> (-19.2151, 2.0706)
  line L58 (-19.2151, 2.0706) -> (-19.4515, 2.162)
  line L59 (-19.4515, 2.162) -> (-19.6863, 2.2657)
  line L60 (-19.6863, 2.2657) -> (-19.9195, 2.3804)
  line L61 (-19.9195, 2.3804) -> (-20.1511, 2.5052)
  line L62 (-20.1511, 2.5052) -> (-20.381, 2.6396)
  line L63 (-20.381, 2.6396) -> (-20.6091, 2.783)
  line L64 (-20.6091, 2.783) -> (-20.8355, 2.9351)
  line L65 (-20.8355, 2.9351) -> (-21.0039, 3.0547)
  line L66 (-21.0039, 3.0547) -> (-20.9199, 3.5854)
  line L67 (-20.9199, 3.5854) -> (-20.7227, 3.6471)
  line L68 (-20.7227, 3.6471) -> (-20.4605, 3.7218)
  line L69 (-20.4605, 3.7218) -> (-20.1992, 3.7876)
  line L70 (-20.1992, 3.7876) -> (-19.939, 3.8444)
  line L71 (-19.939, 3.8444) -> (-19.6802, 3.8916)
  line L72 (-19.6802, 3.8916) -> (-19.4229, 3.9286)
  line L73 (-19.4229, 3.9286) -> (-19.1676, 3.9547)
  line L74 (-19.1676, 3.9547) -> (-18.9145, 3.9685)
  line L75 (-18.9145, 3.9685) -> (-18.7889, 3.9703)
  line L76 (-18.7889, 3.9703) -> (-18.6642, 3.968)
  line L77 (-18.6642, 3.968) -> (-18.5404, 3.9611)
  line L78 (-18.5404, 3.9611) -> (-18.479, 3.9554)
  line L79 (-18.479, 3.9554) -> (-18.418, 3.9479)
  line L80 (-18.418, 3.9479) -> (-18.2968, 4.211)
  line L81 (-18.2968, 4.211) -> (-18.2143, 4.5545)
  line L82 (-18.2143, 4.5545) -> (-18.2028, 4.844)
  line L83 (-18.2028, 4.844) -> (-18.2606, 4.865)
  line L84 (-18.2606, 4.865) -> (-18.3179, 4.8878)
  line L85 (-18.3179, 4.8878) -> (-18.4314, 4.9378)
  line L86 (-18.4314, 4.9378) -> (-18.5435, 4.9924)
  line L87 (-18.5435, 4.9924) -> (-18.6546, 5.051)
  line L88 (-18.6546, 5.051) -> (-18.8738, 5.1783)
  line L89 (-18.8738, 5.1783) -> (-19.0895, 5.3174)
  line L90 (-19.0895, 5.3174) -> (-19.3019, 5.4672)
  line L91 (-19.3019, 5.4672) -> (-19.5111, 5.6267)
  line L92 (-19.5111, 5.6267) -> (-19.7171, 5.7954)
  line L93 (-19.7171, 5.7954) -> (-19.92, 5.9727)
  line L94 (-19.92, 5.9727) -> (-20.1198, 6.1583)
  line L95 (-20.1198, 6.1583) -> (-20.2675, 6.3028)
  line L96 (-20.2675, 6.3028) -> (-20.1014, 6.8139)
  line L97 (-20.1014, 6.8139) -> (-19.897, 6.8439)
  line L98 (-19.897, 6.8439) -> (-19.6263, 6.8767)
  line L99 (-19.6263, 6.8767) -> (-19.358, 6.9009)
  line L100 (-19.358, 6.9009) -> (-19.0921, 6.9162)
  line L101 (-19.0921, 6.9162) -> (-18.8291, 6.9223)
  line L102 (-18.8291, 6.9223) -> (-18.5692, 6.9186)
  line L103 (-18.5692, 6.9186) -> (-18.3129, 6.9044)
  line L104 (-18.3129, 6.9044) -> (-18.0608, 6.8785)
  line L105 (-18.0608, 6.8785) -> (-17.9365, 6.8606)
  line L106 (-17.9365, 6.8606) -> (-17.8137, 6.8389)
  line L107 (-17.8137, 6.8389) -> (-17.6925, 6.8127)
  line L108 (-17.6925, 6.8127) -> (-17.6327, 6.7975)
  line L109 (-17.6327, 6.7975) -> (-17.5737, 6.7805)
  line L110 (-17.5737, 6.7805) -> (-17.4127, 7.0214)
  line L111 (-17.4127, 7.0214) -> (-17.2776, 7.3478)
  line L112 (-17.2776, 7.3478) -> (-17.221, 7.6319)
  line L113 (-17.221, 7.6319) -> (-17.2748, 7.6617)
  line L114 (-17.2748, 7.6617) -> (-17.3278, 7.6932)
  line L115 (-17.3278, 7.6932) -> (-17.432, 7.7603)
  line L116 (-17.432, 7.7603) -> (-17.5342, 7.8318)
  line L117 (-17.5342, 7.8318) -> (-17.6348, 7.907)
  line L118 (-17.6348, 7.907) -> (-17.8314, 8.067)
  line L119 (-17.8314, 8.067) -> (-18.0227, 8.2382)
  line L120 (-18.0227, 8.2382) -> (-18.209, 8.4194)
  line L121 (-18.209, 8.4194) -> (-18.3907, 8.6097)
  line L122 (-18.3907, 8.6097) -> (-18.5678, 8.8085)
  line L123 (-18.5678, 8.8085) -> (-18.7404, 9.0154)
  line L124 (-18.7404, 9.0154) -> (-18.9087, 9.23)
  line L125 (-18.9087, 9.23) -> (-19.032, 9.3957)
  line L126 (-19.032, 9.3957) -> (-18.788, 9.8745)
  line L127 (-18.788, 9.8745) -> (-18.5814, 9.8722)
  line L128 (-18.5814, 9.8722) -> (-18.309, 9.8622)
  line L129 (-18.309, 9.8622) -> (-18.0401, 9.8442)
  line L130 (-18.0401, 9.8442) -> (-17.7751, 9.8177)
  line L131 (-17.7751, 9.8177) -> (-17.5144, 9.7826)
  line L132 (-17.5144, 9.7826) -> (-17.2583, 9.7383)
  line L133 (-17.2583, 9.7383) -> (-17.0074, 9.6842)
  line L134 (-17.0074, 9.6842) -> (-16.7624, 9.6192)
  line L135 (-16.7624, 9.6192) -> (-16.6424, 9.5821)
  line L136 (-16.6424, 9.5821) -> (-16.5245, 9.5414)
  line L137 (-16.5245, 9.5414) -> (-16.4089, 9.4965)
  line L138 (-16.4089, 9.4965) -> (-16.3523, 9.4722)
  line L139 (-16.3523, 9.4722) -> (-16.2966, 9.4461)
  line L140 (-16.2966, 9.4461) -> (-16.1, 9.659)
  line L141 (-16.1, 9.659) -> (-15.9154, 9.9601)
  line L142 (-15.9154, 9.9601) -> (-15.815, 10.2319)
  line L143 (-15.815, 10.2319) -> (-15.8635, 10.2697)
  line L144 (-15.8635, 10.2697) -> (-15.911, 10.3091)
  line L145 (-15.911, 10.3091) -> (-16.0034, 10.3917)
  line L146 (-16.0034, 10.3917) -> (-16.0932, 10.4784)
  line L147 (-16.0932, 10.4784) -> (-16.1807, 10.5684)
  line L148 (-16.1807, 10.5684) -> (-16.3499, 10.7572)
  line L149 (-16.3499, 10.7572) -> (-16.512, 10.9561)
  line L150 (-16.512, 10.9561) -> (-16.6677, 11.1642)
  line L151 (-16.6677, 11.1642) -> (-16.8174, 11.3806)
  line L152 (-16.8174, 11.3806) -> (-16.9612, 11.6047)
  line L153 (-16.9612, 11.6047) -> (-17.0994, 11.836)
  line L154 (-17.0994, 11.836) -> (-17.232, 12.0743)
  line L155 (-17.232, 12.0743) -> (-17.3279, 12.2573)
  line L156 (-17.3279, 12.2573) -> (-17.012, 12.6921)
  line L157 (-17.012, 12.6921) -> (-16.8083, 12.6575)
  line L158 (-16.8083, 12.6575) -> (-16.5408, 12.605)
  line L159 (-16.5408, 12.605) -> (-16.278, 12.545)
  line L160 (-16.278, 12.545) -> (-16.0205, 12.4775)
  line L161 (-16.0205, 12.4775) -> (-15.7684, 12.402)
  line L162 (-15.7684, 12.402) -> (-15.5224, 12.3182)
  line L163 (-15.5224, 12.3182) -> (-15.2831, 12.2255)
  line L164 (-15.2831, 12.2255) -> (-15.0512, 12.123)
  line L165 (-15.0512, 12.123) -> (-14.9386, 12.0675)
  line L166 (-14.9386, 12.0675) -> (-14.8285, 12.0089)
  line L167 (-14.8285, 12.0089) -> (-14.7213, 11.9465)
  line L168 (-14.7213, 11.9465) -> (-14.6692, 11.9136)
  line L169 (-14.6692, 11.9136) -> (-14.6183, 11.8792)
  line L170 (-14.6183, 11.8792) -> (-14.3908, 12.0586)
  line L171 (-14.3908, 12.0586) -> (-14.1614, 12.3272)
  line L172 (-14.1614, 12.3272) -> (-14.0197, 12.58)
  line L173 (-14.0197, 12.58) -> (-14.0617, 12.6249)
  line L174 (-14.0617, 12.6249) -> (-14.1024, 12.6712)
  line L175 (-14.1024, 12.6712) -> (-14.1807, 12.7673)
  line L176 (-14.1807, 12.7673) -> (-14.2559, 12.8669)
  line L177 (-14.2559, 12.8669) -> (-14.3282, 12.9695)
  line L178 (-14.3282, 12.9695) -> (-14.4658, 13.1824)
  line L179 (-14.4658, 13.1824) -> (-14.5948, 13.4043)
  line L180 (-14.5948, 13.4043) -> (-14.7161, 13.6342)
  line L181 (-14.7161, 13.6342) -> (-14.83, 13.8713)
  line L182 (-14.83, 13.8713) -> (-14.937, 14.1151)
  line L183 (-14.937, 14.1151) -> (-15.0373, 14.3653)
  line L184 (-15.0373, 14.3653) -> (-15.131, 14.6213)
  line L185 (-15.131, 14.6213) -> (-15.1971, 14.8171)
  line L186 (-15.1971, 14.8171) -> (-14.8171, 15.1971)
  line L187 (-14.8171, 15.1971) -> (-14.6213, 15.131)
  line L188 (-14.6213, 15.131) -> (-14.3653, 15.0373)
  line L189 (-14.3653, 15.0373) -> (-14.1151, 14.937)
  line L190 (-14.1151, 14.937) -> (-13.8713, 14.83)
  line L191 (-13.8713, 14.83) -> (-13.6342, 14.7161)
  line L192 (-13.6342, 14.7161) -> (-13.4043, 14.5948)
  line L193 (-13.4043, 14.5948) -> (-13.1824, 14.4658)
  line L194 (-13.1824, 14.4658) -> (-12.9695, 14.3282)
  line L195 (-12.9695, 14.3282) -> (-12.8669, 14.2559)
  line L196 (-12.8669, 14.2559) -> (-12.7673, 14.1807)
  line L197 (-12.7673, 14.1807) -> (-12.6713, 14.1024)
  line L198 (-12.6713, 14.1024) -> (-12.6249, 14.0617)
  line L199 (-12.6249, 14.0617) -> (-12.58, 14.0197)
  line L200 (-12.58, 14.0197) -> (-12.3272, 14.1614)
  line L201 (-12.3272, 14.1614) -> (-12.0586, 14.3908)
  line L202 (-12.0586, 14.3908) -> (-11.8792, 14.6183)
  line L203 (-11.8792, 14.6183) -> (-11.9136, 14.6692)
  line L204 (-11.9136, 14.6692) -> (-11.9465, 14.7213)
  line L205 (-11.9465, 14.7213) -> (-12.0089, 14.8285)
  line L206 (-12.0089, 14.8285) -> (-12.0675, 14.9386)
  line L207 (-12.0675, 14.9386) -> (-12.123, 15.0512)
  line L208 (-12.123, 15.0512) -> (-12.2255, 15.2831)
  line L209 (-12.2255, 15.2831) -> (-12.3182, 15.5224)
  line L210 (-12.3182, 15.5224) -> (-12.402, 15.7684)
  line L211 (-12.402, 15.7684) -> (-12.4775, 16.0205)
  line L212 (-12.4775, 16.0205) -> (-12.545, 16.278)
  line L213 (-12.545, 16.278) -> (-12.605, 16.5408)
  line L214 (-12.605, 16.5408) -> (-12.6575, 16.8083)
  line L215 (-12.6575, 16.8083) -> (-12.6921, 17.012)
  line L216 (-12.6921, 17.012) -> (-12.2573, 17.3279)
  line L217 (-12.2573, 17.3279) -> (-12.0743, 17.232)
  line L218 (-12.0743, 17.232) -> (-11.8361, 17.0994)
  line L219 (-11.8361, 17.0994) -> (-11.6047, 16.9612)
  line L220 (-11.6047, 16.9612) -> (-11.3806, 16.8174)
  line L221 (-11.3806, 16.8174) -> (-11.1642, 16.6677)
  line L222 (-11.1642, 16.6677) -> (-10.9562, 16.512)
  line L223 (-10.9562, 16.512) -> (-10.7572, 16.3499)
  line L224 (-10.7572, 16.3499) -> (-10.5684, 16.1807)
  line L225 (-10.5684, 16.1807) -> (-10.4784, 16.0932)
  line L226 (-10.4784, 16.0932) -> (-10.3917, 16.0034)
  line L227 (-10.3917, 16.0034) -> (-10.3092, 15.911)
  line L228 (-10.3092, 15.911) -> (-10.2697, 15.8635)
  line L229 (-10.2697, 15.8635) -> (-10.2319, 15.815)
  line L230 (-10.2319, 15.815) -> (-9.9601, 15.9154)
  line L231 (-9.9601, 15.9154) -> (-9.6589, 16.1)
  line L232 (-9.6589, 16.1) -> (-9.4461, 16.2966)
  line L233 (-9.4461, 16.2966) -> (-9.4722, 16.3523)
  line L234 (-9.4722, 16.3523) -> (-9.4965, 16.4089)
  line L235 (-9.4965, 16.4089) -> (-9.5414, 16.5245)
  line L236 (-9.5414, 16.5245) -> (-9.582, 16.6424)
  line L237 (-9.582, 16.6424) -> (-9.6192, 16.7624)
  line L238 (-9.6192, 16.7624) -> (-9.6842, 17.0074)
  line L239 (-9.6842, 17.0074) -> (-9.7383, 17.2583)
  line L240 (-9.7383, 17.2583) -> (-9.7826, 17.5144)
  line L241 (-9.7826, 17.5144) -> (-9.8177, 17.7751)
  line L242 (-9.8177, 17.7751) -> (-9.8441, 18.0401)
  line L243 (-9.8441, 18.0401) -> (-9.8622, 18.309)
  line L244 (-9.8622, 18.309) -> (-9.8722, 18.5814)
  line L245 (-9.8722, 18.5814) -> (-9.8745, 18.788)
  line L246 (-9.8745, 18.788) -> (-9.3957, 19.032)
  line L247 (-9.3957, 19.032) -> (-9.23, 18.9087)
  line L248 (-9.23, 18.9087) -> (-9.0154, 18.7404)
  line L249 (-9.0154, 18.7404) -> (-8.8085, 18.5678)
  line L250 (-8.8085, 18.5678) -> (-8.6097, 18.3907)
  line L251 (-8.6097, 18.3907) -> (-8.4194, 18.209)
  line L252 (-8.4194, 18.209) -> (-8.2382, 18.0227)
  line L253 (-8.2382, 18.0227) -> (-8.067, 17.8314)
  line L254 (-8.067, 17.8314) -> (-7.907, 17.6348)
  line L255 (-7.907, 17.6348) -> (-7.8318, 17.5342)
  line L256 (-7.8318, 17.5342) -> (-7.7603, 17.432)
  line L257 (-7.7603, 17.432) -> (-7.6932, 17.3278)
  line L258 (-7.6932, 17.3278) -> (-7.6617, 17.2748)
  line L259 (-7.6617, 17.2748) -> (-7.6319, 17.221)
  line L260 (-7.6319, 17.221) -> (-7.3478, 17.2776)
  line L261 (-7.3478, 17.2776) -> (-7.0214, 17.4127)
  line L262 (-7.0214, 17.4127) -> (-6.7805, 17.5736)
  line L263 (-6.7805, 17.5736) -> (-6.7975, 17.6327)
  line L264 (-6.7975, 17.6327) -> (-6.8127, 17.6925)
  line L265 (-6.8127, 17.6925) -> (-6.8389, 17.8137)
  line L266 (-6.8389, 17.8137) -> (-6.8606, 17.9365)
  line L267 (-6.8606, 17.9365) -> (-6.8785, 18.0608)
  line L268 (-6.8785, 18.0608) -> (-6.9044, 18.3129)
  line L269 (-6.9044, 18.3129) -> (-6.9187, 18.5692)
  line L270 (-6.9187, 18.5692) -> (-6.9223, 18.8291)
  line L271 (-6.9223, 18.8291) -> (-6.9162, 19.0921)
  line L272 (-6.9162, 19.0921) -> (-6.9009, 19.358)
  line L273 (-6.9009, 19.358) -> (-6.8767, 19.6263)
  line L274 (-6.8767, 19.6263) -> (-6.8439, 19.897)
  line L275 (-6.8439, 19.897) -> (-6.8139, 20.1014)
  line L276 (-6.8139, 20.1014) -> (-6.3028, 20.2675)
  line L277 (-6.3028, 20.2675) -> (-6.1584, 20.1198)
  line L278 (-6.1584, 20.1198) -> (-5.9728, 19.92)
  line L279 (-5.9728, 19.92) -> (-5.7954, 19.7171)
  line L280 (-5.7954, 19.7171) -> (-5.6267, 19.5111)
  line L281 (-5.6267, 19.5111) -> (-5.4672, 19.3019)
  line L282 (-5.4672, 19.3019) -> (-5.3174, 19.0895)
  line L283 (-5.3174, 19.0895) -> (-5.1783, 18.8738)
  line L284 (-5.1783, 18.8738) -> (-5.051, 18.6546)
  line L285 (-5.051, 18.6546) -> (-4.9925, 18.5435)
  line L286 (-4.9925, 18.5435) -> (-4.9378, 18.4314)
  line L287 (-4.9378, 18.4314) -> (-4.8878, 18.3179)
  line L288 (-4.8878, 18.3179) -> (-4.865, 18.2606)
  line L289 (-4.865, 18.2606) -> (-4.844, 18.2028)
  line L290 (-4.844, 18.2028) -> (-4.5545, 18.2143)
  line L291 (-4.5545, 18.2143) -> (-4.211, 18.2968)
  line L292 (-4.211, 18.2968) -> (-3.9479, 18.418)
  line L293 (-3.9479, 18.418) -> (-3.9554, 18.479)
  line L294 (-3.9554, 18.479) -> (-3.9611, 18.5404)
  line L295 (-3.9611, 18.5404) -> (-3.968, 18.6642)
  line L296 (-3.968, 18.6642) -> (-3.9703, 18.7889)
  line L297 (-3.9703, 18.7889) -> (-3.9685, 18.9145)
  line L298 (-3.9685, 18.9145) -> (-3.9547, 19.1676)
  line L299 (-3.9547, 19.1676) -> (-3.9286, 19.4229)
  line L300 (-3.9286, 19.4229) -> (-3.8916, 19.6802)
  line L301 (-3.8916, 19.6802) -> (-3.8444, 19.939)
  line L302 (-3.8444, 19.939) -> (-3.7876, 20.1992)
  line L303 (-3.7876, 20.1992) -> (-3.7218, 20.4605)
  line L304 (-3.7218, 20.4605) -> (-3.6471, 20.7227)
  line L305 (-3.6471, 20.7227) -> (-3.5854, 20.9199)
  line L306 (-3.5854, 20.9199) -> (-3.0547, 21.0039)
  line L307 (-3.0547, 21.0039) -> (-2.9351, 20.8355)
  line L308 (-2.9351, 20.8355) -> (-2.783, 20.6091)
  line L309 (-2.783, 20.6091) -> (-2.6396, 20.381)
  line L310 (-2.6396, 20.381) -> (-2.5053, 20.1511)
  line L311 (-2.5053, 20.1511) -> (-2.3804, 19.9195)
  line L312 (-2.3804, 19.9195) -> (-2.2657, 19.6863)
  line L313 (-2.2657, 19.6863) -> (-2.162, 19.4515)
  line L314 (-2.162, 19.4515) -> (-2.0706, 19.2151)
  line L315 (-2.0706, 19.2151) -> (-2.0301, 19.0962)
  line L316 (-2.0301, 19.0962) -> (-1.9937, 18.9769)
  line L317 (-1.9937, 18.9769) -> (-1.9621, 18.857)
  line L318 (-1.9621, 18.857) -> (-1.9485, 18.7969)
  line L319 (-1.9485, 18.7969) -> (-1.9368, 18.7365)
  line L320 (-1.9368, 18.7365) -> (-1.6491, 18.7025)
  line L321 (-1.6491, 18.7025) -> (-1.297, 18.7302)
  line L322 (-1.297, 18.7302) -> (-1.018, 18.8088)
  line L323 (-1.018, 18.8088) -> (-1.016, 18.8703)
  line L324 (-1.016, 18.8703) -> (-1.012, 18.9318)
  line L325 (-1.012, 18.9318) -> (-0.9995, 19.0551)
  line L326 (-0.9995, 19.0551) -> (-0.9822, 19.1787)
  line L327 (-0.9822, 19.1787) -> (-0.9608, 19.3024)
  line L328 (-0.9608, 19.3024) -> (-0.9075, 19.5502)
  line L329 (-0.9075, 19.5502) -> (-0.8418, 19.7984)
  line L330 (-0.8418, 19.7984) -> (-0.765, 20.0467)
  line L331 (-0.765, 20.0467) -> (-0.6779, 20.2949)
  line L332 (-0.6779, 20.2949) -> (-0.5812, 20.543)
  line L333 (-0.5812, 20.543) -> (-0.4752, 20.7908)
  line L334 (-0.4752, 20.7908) -> (-0.3604, 21.0381)
  line L335 (-0.3604, 21.0381) -> (-0.2687, 21.2232)
  line L336 (-0.2687, 21.2232) -> (0.2687, 21.2232)
  line L337 (0.2687, 21.2232) -> (0.3604, 21.0381)
  line L338 (0.3604, 21.0381) -> (0.4752, 20.7908)
  line L339 (0.4752, 20.7908) -> (0.5812, 20.543)
  line L340 (0.5812, 20.543) -> (0.6779, 20.2949)
  line L341 (0.6779, 20.2949) -> (0.765, 20.0467)
  line L342 (0.765, 20.0467) -> (0.8418, 19.7984)
  line L343 (0.8418, 19.7984) -> (0.9075, 19.5502)
  line L344 (0.9075, 19.5502) -> (0.9608, 19.3024)
  line L345 (0.9608, 19.3024) -> (0.9822, 19.1787)
  line L346 (0.9822, 19.1787) -> (0.9995, 19.0551)
  line L347 (0.9995, 19.0551) -> (1.012, 18.9318)
  line L348 (1.012, 18.9318) -> (1.016, 18.8703)
  line L349 (1.016, 18.8703) -> (1.018, 18.8088)
  line L350 (1.018, 18.8088) -> (1.2969, 18.7302)
  line L351 (1.2969, 18.7302) -> (1.6491, 18.7025)
  line L352 (1.6491, 18.7025) -> (1.9368, 18.7365)
  line L353 (1.9368, 18.7365) -> (1.9485, 18.7969)
  line L354 (1.9485, 18.7969) -> (1.9621, 18.857)
  line L355 (1.9621, 18.857) -> (1.9937, 18.9769)
  line L356 (1.9937, 18.9769) -> (2.0301, 19.0962)
  line L357 (2.0301, 19.0962) -> (2.0706, 19.2151)
  line L358 (2.0706, 19.2151) -> (2.162, 19.4515)
  line L359 (2.162, 19.4515) -> (2.2657, 19.6863)
  line L360 (2.2657, 19.6863) -> (2.3804, 19.9195)
  line L361 (2.3804, 19.9195) -> (2.5052, 20.1511)
  line L362 (2.5052, 20.1511) -> (2.6396, 20.381)
  line L363 (2.6396, 20.381) -> (2.783, 20.6091)
  line L364 (2.783, 20.6091) -> (2.9351, 20.8354)
  line L365 (2.9351, 20.8354) -> (3.0547, 21.0039)
  line L366 (3.0547, 21.0039) -> (3.5854, 20.9199)
  line L367 (3.5854, 20.9199) -> (3.6471, 20.7227)
  line L368 (3.6471, 20.7227) -> (3.7218, 20.4605)
  line L369 (3.7218, 20.4605) -> (3.7876, 20.1992)
  line L370 (3.7876, 20.1992) -> (3.8444, 19.939)
  line L371 (3.8444, 19.939) -> (3.8916, 19.6802)
  line L372 (3.8916, 19.6802) -> (3.9286, 19.4229)
  line L373 (3.9286, 19.4229) -> (3.9547, 19.1676)
  line L374 (3.9547, 19.1676) -> (3.9685, 18.9145)
  line L375 (3.9685, 18.9145) -> (3.9703, 18.7889)
  line L376 (3.9703, 18.7889) -> (3.968, 18.6642)
  line L377 (3.968, 18.6642) -> (3.9611, 18.5404)
  line L378 (3.9611, 18.5404) -> (3.9554, 18.479)
  line L379 (3.9554, 18.479) -> (3.9479, 18.418)
  line L380 (3.9479, 18.418) -> (4.211, 18.2968)
  line L381 (4.211, 18.2968) -> (4.5545, 18.2143)
  line L382 (4.5545, 18.2143) -> (4.844, 18.2028)
  line L383 (4.844, 18.2028) -> (4.865, 18.2606)
  line L384 (4.865, 18.2606) -> (4.8878, 18.3179)
  line L385 (4.8878, 18.3179) -> (4.9378, 18.4313)
  line L386 (4.9378, 18.4313) -> (4.9924, 18.5435)
  line L387 (4.9924, 18.5435) -> (5.051, 18.6546)
  line L388 (5.051, 18.6546) -> (5.1783, 18.8738)
  line L389 (5.1783, 18.8738) -> (5.3174, 19.0895)
  line L390 (5.3174, 19.0895) -> (5.4672, 19.3019)
  line L391 (5.4672, 19.3019) -> (5.6267, 19.5111)
  line L392 (5.6267, 19.5111) -> (5.7954, 19.7171)
  line L393 (5.7954, 19.7171) -> (5.9727, 19.92)
  line L394 (5.9727, 19.92) -> (6.1583, 20.1198)
  line L395 (6.1583, 20.1198) -> (6.3028, 20.2675)
  line L396 (6.3028, 20.2675) -> (6.8139, 20.1014)
  line L397 (6.8139, 20.1014) -> (6.8439, 19.897)
  line L398 (6.8439, 19.897) -> (6.8767, 19.6263)
  line L399 (6.8767, 19.6263) -> (6.9009, 19.358)
  line L400 (6.9009, 19.358) -> (6.9162, 19.0921)
  line L401 (6.9162, 19.0921) -> (6.9223, 18.8291)
  line L402 (6.9223, 18.8291) -> (6.9186, 18.5692)
  line L403 (6.9186, 18.5692) -> (6.9044, 18.3129)
  line L404 (6.9044, 18.3129) -> (6.8785, 18.0608)
  line L405 (6.8785, 18.0608) -> (6.8606, 17.9365)
  line L406 (6.8606, 17.9365) -> (6.8389, 17.8137)
  line L407 (6.8389, 17.8137) -> (6.8127, 17.6925)
  line L408 (6.8127, 17.6925) -> (6.7975, 17.6327)
  line L409 (6.7975, 17.6327) -> (6.7804, 17.5736)
  line L410 (6.7804, 17.5736) -> (7.0214, 17.4127)
  line L411 (7.0214, 17.4127) -> (7.3478, 17.2776)
  line L412 (7.3478, 17.2776) -> (7.6319, 17.221)
  line L413 (7.6319, 17.221) -> (7.6617, 17.2748)
  line L414 (7.6617, 17.2748) -> (7.6932, 17.3278)
  line L415 (7.6932, 17.3278) -> (7.7603, 17.432)
  line L416 (7.7603, 17.432) -> (7.8318, 17.5342)
  line L417 (7.8318, 17.5342) -> (7.907, 17.6348)
  line L418 (7.907, 17.6348) -> (8.067, 17.8314)
  line L419 (8.067, 17.8314) -> (8.2382, 18.0227)
  line L420 (8.2382, 18.0227) -> (8.4194, 18.209)
  line L421 (8.4194, 18.209) -> (8.6097, 18.3907)
  line L422 (8.6097, 18.3907) -> (8.8085, 18.5678)
  line L423 (8.8085, 18.5678) -> (9.0154, 18.7404)
  line L424 (9.0154, 18.7404) -> (9.23, 18.9087)
  line L425 (9.23, 18.9087) -> (9.3957, 19.032)
  line L426 (9.3957, 19.032) -> (9.8745, 18.788)
  line L427 (9.8745, 18.788) -> (9.8722, 18.5815)
  line L428 (9.8722, 18.5815) -> (9.8622, 18.309)
  line L429 (9.8622, 18.309) -> (9.8441, 18.0401)
  line L430 (9.8441, 18.0401) -> (9.8177, 17.7751)
  line L431 (9.8177, 17.7751) -> (9.7826, 17.5144)
  line L432 (9.7826, 17.5144) -> (9.7383, 17.2583)
  line L433 (9.7383, 17.2583) -> (9.6842, 17.0074)
  line L434 (9.6842, 17.0074) -> (9.6192, 16.7624)
  line L435 (9.6192, 16.7624) -> (9.582, 16.6424)
  line L436 (9.582, 16.6424) -> (9.5414, 16.5245)
  line L437 (9.5414, 16.5245) -> (9.4965, 16.4089)
  line L438 (9.4965, 16.4089) -> (9.4722, 16.3523)
  line L439 (9.4722, 16.3523) -> (9.4461, 16.2966)
  line L440 (9.4461, 16.2966) -> (9.6589, 16.1)
  line L441 (9.6589, 16.1) -> (9.9601, 15.9154)
  line L442 (9.9601, 15.9154) -> (10.2319, 15.815)
  line L443 (10.2319, 15.815) -> (10.2697, 15.8635)
  line L444 (10.2697, 15.8635) -> (10.3091, 15.911)
  line L445 (10.3091, 15.911) -> (10.3917, 16.0034)
  line L446 (10.3917, 16.0034) -> (10.4784, 16.0932)
  line L447 (10.4784, 16.0932) -> (10.5684, 16.1807)
  line L448 (10.5684, 16.1807) -> (10.7572, 16.3499)
  line L449 (10.7572, 16.3499) -> (10.9561, 16.512)
  line L450 (10.9561, 16.512) -> (11.1642, 16.6677)
  line L451 (11.1642, 16.6677) -> (11.3806, 16.8174)
  line L452 (11.3806, 16.8174) -> (11.6047, 16.9612)
  line L453 (11.6047, 16.9612) -> (11.836, 17.0994)
  line L454 (11.836, 17.0994) -> (12.0743, 17.232)
  line L455 (12.0743, 17.232) -> (12.2573, 17.3279)
  line L456 (12.2573, 17.3279) -> (12.6921, 17.012)